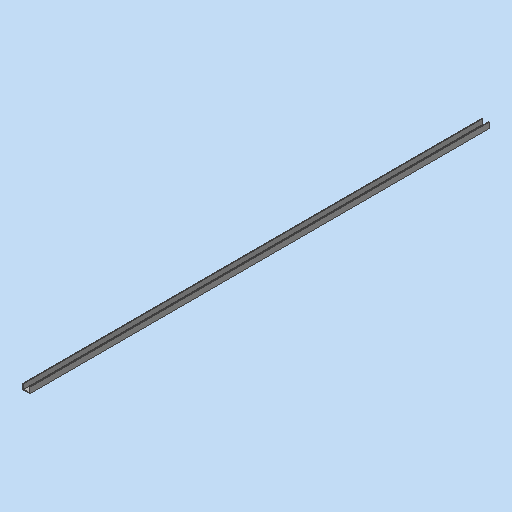
# Autodesk Inventor part: U-Profil PanelSupport 10x8x660mm
Saved by Autodesk Inventor 2023.2 (Build 272271000, 271)
## iProperties
Created: 2023-12-14
Part Number: U-Profil PanelSupport 10x8x660mm
Material: Generisch
Document SubType Name: Modeling
Designer: Nils Bade
Density: 1 g/cm^3
Appearance: Elox-Alu
Description: Nicht vorbestellen, bauhaus
Auf Bestellliste: True
Listed: False
Author: Nils Bade
Autodesk Inventor part; units mm, degrees
ref_plane "YZ Plane" through (0, 0, 0) normal (1, 0, 0) x (0, 1, 0)
ref_plane "XY Plane" through (0, 0, 0) normal (0, 0, 1) x (1, 0, 0)
sketch "Skizze1" plane through (0, 0, 0) normal (0, 0, 1) x (1, 0, 0)
  line L0 (0, 0) -> (5, 0)
  line L1 (5, 0) -> (5, 8)
  line L2 (5, 8) -> (4, 8)
  line L3 (4, 8) -> (4, 1)
  line L4 (4, 1) -> (0, 1)
  line L5 (0, 9.6) -> (0, -1.6) construction
  line L6 (0, 0) -> (-5, 0)
  line L7 (-5, 0) -> (-5, 8)
  line L8 (-5, 8) -> (-4, 8)
  line L9 (-4, 8) -> (-4, 1)
  line L10 (-4, 1) -> (0, 1)
  dimension "d0" = 1
  dimension "d1" = 1
  dimension "d2" = 8
  dimension "d3" = 5
  constraints: 20 end point, 4 perpendicular, 4 symmetric about line, 1 horizontal
  measures "d0" distance between parallel lines of L0 L4
  measures "d1" distance between parallel lines of L3 L1
  measures "d2" distance between parallel lines of L0 L2
  measures "d3" distance of L0.start L0.end
extrude "Ex-UProfil" add sketch "Skizze1" along normal blind 660
sketch "Skizze2" plane through (0, 0, 0) normal (0, 1, 0) x (-1, 0, 0)
  line L0 (5, 0) -> (-5, 0) projected
  line L1 (-5, 0) -> (-5, 660) projected
  line L2 (5, 660) -> (-5, 660) projected
  line L3 (5, 0) -> (5, 660) projected
  line L4 (0, -53) -> (0, 318) construction
  circle A0 centre (0, 650) radius 2.15 construction
  line L5 (0, 651) -> (0, 649) construction
  line L6 (-2.15, 651) -> (-2.15, 649)
  line L7 (2.15, 649) -> (2.15, 651)
  arc A1 (2.15, 651) -> (-2.15, 651) centre (0, 651) ccw
  arc A2 (-2.15, 649) -> (2.15, 649) centre (0, 649) ccw
  circle A3 centre (0, 570) radius 2.15 construction
  line L8 (0, 571) -> (0, 569) construction
  line L9 (-2.15, 571) -> (-2.15, 569)
  line L10 (2.15, 569) -> (2.15, 571)
  arc A4 (2.15, 571) -> (-2.15, 571) centre (0, 571) ccw
  arc A5 (-2.15, 569) -> (2.15, 569) centre (0, 569) ccw
  circle A6 centre (0, 490) radius 2.15 construction
  line L11 (0, 491) -> (0, 489) construction
  line L12 (-2.15, 491) -> (-2.15, 489)
  line L13 (2.15, 489) -> (2.15, 491)
  arc A7 (2.15, 491) -> (-2.15, 491) centre (0, 491) ccw
  arc A8 (-2.15, 489) -> (2.15, 489) centre (0, 489) ccw
  circle A9 centre (0, 410) radius 2.15 construction
  line L14 (0, 411) -> (0, 409) construction
  line L15 (-2.15, 411) -> (-2.15, 409)
  line L16 (2.15, 409) -> (2.15, 411)
  arc A10 (2.15, 411) -> (-2.15, 411) centre (0, 411) ccw
  arc A11 (-2.15, 409) -> (2.15, 409) centre (0, 409) ccw
  circle A12 centre (0, 330) radius 2.15 construction
  line L17 (0, 331) -> (0, 329) construction
  line L18 (-2.15, 331) -> (-2.15, 329)
  line L19 (2.15, 329) -> (2.15, 331)
  arc A13 (2.15, 331) -> (-2.15, 331) centre (0, 331) ccw
  arc A14 (-2.15, 329) -> (2.15, 329) centre (0, 329) ccw
  circle A15 centre (0, 250) radius 2.15 construction
  line L20 (0, 251) -> (0, 249) construction
  line L21 (-2.15, 251) -> (-2.15, 249)
  line L22 (2.15, 249) -> (2.15, 251)
  arc A16 (2.15, 251) -> (-2.15, 251) centre (0, 251) ccw
  arc A17 (-2.15, 249) -> (2.15, 249) centre (0, 249) ccw
  circle A18 centre (0, 170) radius 2.15 construction
  line L23 (0, 171) -> (0, 169) construction
  line L24 (-2.15, 171) -> (-2.15, 169)
  line L25 (2.15, 169) -> (2.15, 171)
  arc A19 (2.15, 171) -> (-2.15, 171) centre (0, 171) ccw
  arc A20 (-2.15, 169) -> (2.15, 169) centre (0, 169) ccw
  circle A21 centre (0, 90) radius 2.15 construction
  line L26 (0, 91) -> (0, 89) construction
  line L27 (-2.15, 91) -> (-2.15, 89)
  line L28 (2.15, 89) -> (2.15, 91)
  arc A22 (2.15, 91) -> (-2.15, 91) centre (0, 91) ccw
  arc A23 (-2.15, 89) -> (2.15, 89) centre (0, 89) ccw
  circle A24 centre (0, 10) radius 2.15 construction
  line L29 (0, 11) -> (0, 9) construction
  line L30 (-2.15, 11) -> (-2.15, 9)
  line L31 (2.15, 9) -> (2.15, 11)
  arc A25 (2.15, 11) -> (-2.15, 11) centre (0, 11) ccw
  arc A26 (-2.15, 9) -> (2.15, 9) centre (0, 9) ccw
  point P0 (0, 0)
  point P1 (0, 653.15)
  point P2 (0, 646.85)
  point P3 (0, 573.15)
  point P4 (0, 566.85)
  point P5 (0, 493.15)
  point P6 (0, 486.85)
  point P7 (0, 413.15)
  point P8 (0, 406.85)
  point P9 (0, 333.15)
  point P10 (0, 326.85)
  point P11 (0, 253.15)
  point P12 (0, 246.85)
  point P13 (0, 173.15)
  point P14 (0, 166.85)
  point P15 (0, 93.15)
  point P16 (0, 86.85)
  point P17 (0, 13.15)
  point P18 (0, 6.85)
  dimension "d6" = 4.3
  dimension "d7" = 10
  dimension "d8" = 4.3
  dimension "d9" = 6.3
  dimension "d21" = 80
  constraints: 72 end point, 38 point on circle, 27 centre point, 4 tangent, 2 point on line, 1 midpoint, 1 parallel, 1 vertical, 120 other
  measures "d6" diameter of A0
  measures "d7" distance from line of L2 A0.centre
  measures "d8" diameter of A2
  measures "d9" distance of point (0, 653.15) point (0, 646.85)
  measures "d21" distance of A0.centre A3.centre
extrude "Ex-Bohrungen" cut sketch "Skizze2" along normal up to surface (1 mm away) contours A1 L7 A2 L6 | A4 L10 A5 L9 | A7 L13 A8 L12 | A10 L16 A11 L15 | A13 L19 A14 L18 | A16 L22 A17 L21 | A19 L25 A20 L24 | A22 L28 A23 L27 | A25 L31 A26 L30
equation "\"d8\" = d6"
